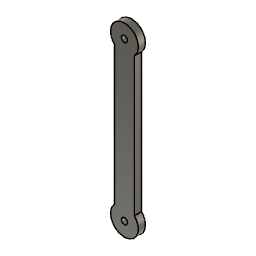
new link v3 (Autodesk Fusion 360 design; units mm, degrees)
Autodesk Fusion 360 part; units mm, degrees
sketch "Sketch1" plane through (0, 0, 0) normal (0, 1, 0) x (1, 0, 0)
  line L0 (-5, 29.899) -> (-5, -40.101)
  line L1 (5, -40.101) -> (5, 29.899)
  circle A0 centre (0, -45) radius 1.55
  arc A1 (-5, -40.101) -> (5, -40.101) centre (0, -45) ccw
  arc A2 (5, 29.899) -> (-5, 29.899) centre (0, 34.798) ccw
  circle A3 centre (0, 34.798) radius 1.55
  dimension "d3" = 3.1
  dimension "d4" = 14
  dimension "d7" = 70
  dimension "d8" = 7
  dimension "d9" = 3.1
  constraint parallel L0 L1
  constraint concentric A0 A1
  constraint coincident A2.centre A3.centre
  measures "d3" diameter of A0
  measures "d4" diameter of A1
  measures "d7" distance of L1.start L1.end
  measures "d8" radius of A2
  measures "d9" diameter of A3
extrude "Extrude1" add sketch "Sketch1" along normal blind 5
sketch "Sketch2" plane through (0, 0, 0) normal (0, -1, 0) x (1, 0, 0)
  circle A0 centre (0, -34.798) radius 1.55
  circle A1 centre (0, 45) radius 1.55
  arc A2 (-5, -29.899) -> (5, -29.899) centre (0, -34.798) ccw
  line L0 (5, -29.899) -> (5, 40.101)
  arc A3 (5, 40.101) -> (-5, 40.101) centre (0, 45) ccw
  line L1 (-5, 40.101) -> (-5, -29.899)
extrude "Extrude2" cut sketch "Sketch2" against normal blind 1
extrude "Extrude3" cut 1 faces at (-1.6667, 1, 16.7677) along direction (0, 1, 0) blind 0.4
